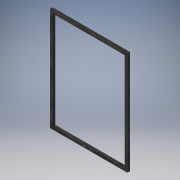
# Autodesk Inventor part: Steel support4
Saved by Autodesk Inventor 2019 (Build 230136000, 136)
## iProperties
Created: 2021-03-08
Part Number: Steel support4
Material: Steel
Document SubType Name: Modeling
Designer: User
Density: 7.85 g/cm^3
Appearance: Plate
Author: User
Autodesk Inventor part; units mm, degrees
ref_plane "YZ Plane" through (0, 0, 0) normal (1, 0, 0) x (0, 1, 0)
ref_plane "XZ Plane" through (0, 0, 0) normal (0, 1, 0) x (-1, 0, 0)
ref_plane "XY Plane" through (0, 0, 0) normal (0, 0, 1) x (1, 0, 0)
sketch "Sketch1" plane through (0, 0, 0) normal (0, 0, 1) x (1, 0, 0)
  line L0 (-127.5, 275) -> (172.5, 275)
  line L1 (172.5, 275) -> (172.5, -125)
  line L2 (172.5, -125) -> (-127.5, -125)
  line L3 (-127.5, -125) -> (-127.5, 275)
  line L4 (-117.5, 265) -> (162.5, 265)
  line L5 (162.5, 265) -> (162.5, -115)
  line L6 (162.5, -115) -> (-117.5, -115)
  line L7 (-117.5, -115) -> (-117.5, 265)
  point P0 (0, 0)
  dimension "d0" = 300
  dimension "d1" = 10
  dimension "d2" = 10
  dimension "d3" = 10
  dimension "d4" = 10
  dimension "d5" = 400
  dimension "d6" = 172.5
  dimension "d7" = 115
  constraints: 16 end point, 4 parallel, 2 horizontal, 2 perpendicular
  measures "d0" distance between parallel lines of L1 L3
  measures "d1" distance between parallel lines of L1 L5
  measures "d2" distance between parallel lines of L6 L2
  measures "d3" distance between parallel lines of L7 L3
  measures "d4" distance between parallel lines of L4 L0
  measures "d5" distance between parallel lines of L0 L2
  measures "d6" distance from line of point (0, 0) L1
  measures "d7" distance from line of point (0, 0) L6
extrude "Extrusion1" add sketch "Sketch1" along normal mid plane 10
body "Solid1"
